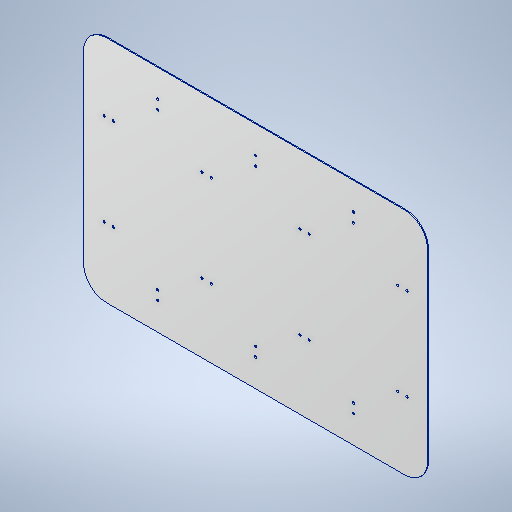
# Autodesk Inventor part: plate2mm
Saved by Autodesk Inventor 2025 (Build 290162000, 162)
## iProperties
Created: 2025-09-29
Part Number: plate2mm
Material: Aluminum 6061
Document SubType Name: Sheet Metal
Designer: hp
Density: 2.7 g/cm^3
Appearance: Aluminum - Flat
Mass: 2145.65 g
Surface Area: 8005.32 cm^2
Volume: 794.687 cm^3
Sheet Metal Rule: Default_mm
Author: hp
Autodesk Inventor part; units mm, degrees
ref_plane "YZ Plane" through (0, 0, 0) normal (1, 0, 0) x (0, 1, 0)
ref_plane "XZ Plane" through (0, 0, 0) normal (0, 1, 0) x (-1, 0, 0)
ref_plane "XY Plane" through (0, 0, 0) normal (0, 0, 1) x (1, 0, 0)
sketch "Sketch1" plane through (0, 0, 0) normal (0, 0, 1) x (1, 0, 0)
  line L0 (-325, 250) -> (325, 250)
  line L1 (375, 200) -> (375, -200)
  line L2 (325, -250) -> (-325, -250)
  line L3 (-375, -200) -> (-375, 200)
  line L4 (-375, 250) -> (375, -250) construction
  line L5 (375, 250) -> (-375, -250) construction
  arc A0 (-325, 250) -> (-375, 200) centre (-325, 200) ccw
  arc A1 (-375, -200) -> (-325, -250) centre (-325, -200) ccw
  arc A2 (375, 200) -> (325, 250) centre (325, 200) ccw
  arc A3 (325, -250) -> (375, -200) centre (325, -200) ccw
  point P0 (0, 0)
  dimension "d0" = 750
  dimension "d1" = 500
  dimension "d2" = 50
  constraints: 12 end point, 8 point on circle, 8 point on line, 8 tangent, 4 centre point, 3 equal radius, 2 midpoint, 2 parallel, 1 horizontal, 1 perpendicular
  measures "d0" distance of L4.end L5.end
  measures "d1" distance of L5.start L4.end
  measures "d2" radius of A0
extrude "Extrusion1" add sketch "Sketch1" along normal blind 2
sketch "Sketch2" plane through (0, 0, 2) normal (0, 0, 1) x (1, 0, 0)
  line L0 (-340, 200) -> (340, 200)
  line L1 (340, 200) -> (340, -200)
  line L2 (340, -200) -> (-340, -200)
  line L3 (-340, -200) -> (-340, 200)
  line L4 (-340, 200) -> (340, -200) construction
  line L5 (340, 200) -> (-340, -200) construction
  line L6 (300, 160) -> (-300, 160)
  line L7 (-300, 160) -> (-300, -160)
  line L8 (-300, -160) -> (300, -160)
  line L9 (300, -160) -> (300, 160)
  line L10 (300, 160) -> (126.67, 160)
  line L11 (126.67, 160) -> (126.67, -160)
  line L12 (126.67, -160) -> (300, -160)
  line L13 (300, -160) -> (300, 160)
  line L14 (-300, 160) -> (-126.67, 160)
  line L15 (-126.67, 160) -> (-126.67, -160)
  line L16 (-126.67, -160) -> (-300, -160)
  line L17 (-300, -160) -> (-300, 160)
  line L18 (-86.67, -160) -> (86.67, -160)
  line L19 (86.67, -160) -> (86.67, 160)
  line L20 (86.67, 160) -> (-86.67, 160)
  line L21 (-86.67, 160) -> (-86.67, -160)
  line L22 (-86.67, -160) -> (86.67, 160) construction
  line L23 (86.67, -160) -> (-86.67, 160) construction
  line L24 (-96.67, 160) -> (-96.67, -160)
  line L25 (-116.67, 160) -> (-116.67, -160)
  line L26 (116.67, 160) -> (116.67, -160)
  line L27 (96.67, 160) -> (96.67, -160)
  line L28 (330, 190) -> (-330, 190)
  line L29 (-330, 190) -> (-330, -190)
  line L30 (-330, -190) -> (330, -190)
  line L31 (330, -190) -> (330, 190)
  line L32 (-310, 170) -> (310, 170)
  line L33 (310, 170) -> (310, -170)
  line L34 (310, -170) -> (-310, -170)
  line L35 (-310, -170) -> (-310, 170)
  circle A0 centre (0, -170) radius 2.5
  circle A1 centre (0, -190) radius 2.5
  circle A2 centre (0, 170) radius 2.5
  circle A3 centre (0, 190) radius 2.5
  circle A4 centre (-213.335, 190) radius 2.5
  circle A5 centre (-213.335, 170) radius 2.5
  circle A6 centre (-310, 100) radius 2.5
  circle A7 centre (-330, 100) radius 2.5
  circle A8 centre (-330, -100) radius 2.5
  circle A9 centre (-310, -100) radius 2.5
  circle A10 centre (-213.335, -170) radius 2.5
  circle A11 centre (-213.335, -190) radius 2.5
  circle A12 centre (213.335, 170) radius 2.5
  circle A13 centre (213.335, 190) radius 2.5
  circle A14 centre (213.335, -170) radius 2.5
  circle A15 centre (213.335, -190) radius 2.5
  circle A16 centre (310, 100) radius 2.5
  circle A17 centre (330, 100) radius 2.5
  circle A18 centre (310, -100) radius 2.5
  circle A19 centre (330, -100) radius 2.5
  circle A20 centre (-116.67, 100) radius 2.5
  circle A21 centre (-96.67, 100) radius 2.5
  circle A22 centre (96.67, 100) radius 2.5
  circle A23 centre (116.67, 100) radius 2.5
  circle A24 centre (-116.67, -100) radius 2.5
  circle A25 centre (-96.67, -100) radius 2.5
  circle A26 centre (96.67, -100) radius 2.5
  circle A27 centre (116.67, -100) radius 2.5
  point P0 (0, 0)
  dimension "d5" = 680
  dimension "d6" = 400
  dimension "d15" = 173.33
  dimension "d16" = 173.33
  dimension "d17" = 173.34
  dimension "d18" = 10
  dimension "d19" = 10
  dimension "d20" = 10
  dimension "d21" = 10
  dimension "d22" = 320
  dimension "d23" = 160
  dimension "d24" = 300
  dimension "d25" = 40
  dimension "d26" = 10
  dimension "d27" = 20
  dimension "d28" = 5
  dimension "d29" = 5
  dimension "d30" = 5
  dimension "d31" = 5
  dimension "d32" = 5
  dimension "d33" = 5
  dimension "d34" = 5
  dimension "d35" = 5
  dimension "d36" = 5
  dimension "d37" = 5
  dimension "d38" = 5
  dimension "d39" = 5
  dimension "d40" = 5
  dimension "d41" = 5
  dimension "d42" = 5
  dimension "d43" = 5
  dimension "d44" = 5
  dimension "d45" = 5
  dimension "d46" = 5
  dimension "d47" = 5
  dimension "d48" = 233.33
  dimension "d49" = 193.33
  dimension "d50" = 193.33
  dimension "d51" = 233.33
  dimension "d52" = 233.33
  dimension "d53" = 193.33
  dimension "d54" = 233.33
  dimension "d55" = 193.33
  dimension "d56" = 60
  dimension "d57" = 60
  dimension "d58" = 60
  dimension "d59" = 60
  dimension "d60" = 60
  dimension "d61" = 60
  dimension "d62" = 60
  dimension "d63" = 60
  dimension "d64" = 5
  dimension "d65" = 5
  dimension "d66" = 5
  dimension "d67" = 5
  dimension "d68" = 5
  dimension "d69" = 5
  dimension "d70" = 5
  dimension "d71" = 5
  dimension "d72" = 60
  dimension "d73" = 60
  dimension "d74" = 60
  dimension "d75" = 60
  dimension "d76" = 60
  constraints: 72 end point, 35 point on line, 28 centre point, 14 parallel, 11 perpendicular, 8 midpoint, 4 horizontal, 6 other
  measures "d5" distance of L1.end L2.end
  measures "d6" distance of L0.end L1.end
  measures "d15" distance of L12.end L11.end
  measures "d16" distance of L15.end L16.end
  measures "d17" distance of L20.end L19.end
  measures "d18" distance between parallel lines of L11 L26
  measures "d19" distance between parallel lines of L19 L27
  measures "d20" distance between parallel lines of L15 L25
  measures "d21" distance between parallel lines of L21 L24
  measures "d22" distance between parallel lines of L8 L6
  measures "d23" distance from line of point (0, 0) L20
  measures "d24" distance from line of point (0, 0) L7
  measures "d25" distance between parallel lines of L19 L11
  measures "d26" distance between parallel lines of L0 L28
  measures "d27" distance between parallel lines of L28 L32
  measures "d28" diameter of A0
  measures "d29" diameter of A1
  measures "d30" diameter of A2
  measures "d31" diameter of A3
  measures "d32" diameter of A4
  measures "d33" diameter of A5
  measures "d34" diameter of A6
  measures "d35" diameter of A7
  measures "d36" diameter of A8
  measures "d37" diameter of A9
  measures "d38" diameter of A10
  measures "d39" diameter of A11
  measures "d40" diameter of A12
  measures "d41" diameter of A13
  measures "d42" diameter of A14
  measures "d43" diameter of A15
  measures "d44" diameter of A16
  measures "d45" diameter of A17
  measures "d46" diameter of A18
  measures "d47" diameter of A19
  measures "d48" diameter of A4.centre L29
  measures "d49" diameter of A5.centre L35
  measures "d50" diameter of A10.centre L35
  measures "d51" diameter of A11.centre L29
  measures "d52" diameter of A15.centre L31
  measures "d53" diameter of A14.centre L33
  measures "d54" diameter of A13.centre L31
  measures "d55" diameter of A12.centre L33
  measures "d56" distance from line of L12 A18.centre
  measures "d57" distance from line of L8 A19.centre
  measures "d58" distance from line of L6 A17.centre
  measures "d59" distance from line of L10 A16.centre
  measures "d60" distance from line of A6.centre L14
  measures "d61" distance from line of L6 A7.centre
  measures "d62" distance from line of L8 A9.centre
  measures "d63" distance from line of L8 A8.centre
  measures "d64" diameter of A20
  measures "d65" diameter of A21
  measures "d66" diameter of A22
  measures "d67" diameter of A23
  measures "d68" diameter of A24
  measures "d69" diameter of A25
  measures "d70" diameter of A26
  measures "d71" diameter of A27
  measures "d72" distance from line of A20.centre L6
  measures "d73" distance from line of L6 A21.centre
  measures "d74" distance from line of L16 A24.centre
  measures "d75" distance from line of L8 A25.centre
  measures "d76" distance from line of A22.centre L6
extrude "Extrusion2" cut sketch "Sketch2" against normal through all contours A23 L26 | L26 A23 | A22 L27 | L27 A22 | A27 L26 | L26 A27 | A26 L27 | L27 A26 | A21 L24 | L24 A21 | A20 L25 | L25 A20 | A25 L24 | L24 A25 | A24 L25 | L25 A24 | A13 L28 | L28 A13 | A17 L31 | L31 A17 | A3 L28 | L28 A3 | A19 L31 | L31 A19 | A4 L28 | L28 A4 | A15 L30 | L30 A15 | A7 L29 | L29 A7 | A1 L30 | L30 A1 | A8 L29 | L29 A8 | A11 L30 | L30 A11 | A12 L32 | L32 A12 | A16 L33 | L33 A16 | A2 L32 | L32 A2 | A18 L33 | L33 A18 | A5 L32 | L32 A5 | A14 L34 | L34 A14 | A6 L35 | L35 A6 | A0 L34 | L34 A0 | A9 L35 | L35 A9 | A10 L34 | L34 A10
equation "\"BendRadius\" = Thickness"
equation "\"BendReliefWidth\" = Thickness"
equation "\"BendReliefDepth\" = 0.5 * Thickness"
equation "\"CornerReliefSize\" = 4 * Thickness"
equation "\"MinimumRemnant\" = 2 * Thickness"
equation "\"TransitionRadius\" = BendRadius"
equation "\"JacobiRadiusSize\" = BendRadius"
equation "\"GapSize\" = Thickness"
equation "\"Thickness\" = 2"
body "Solid1"
